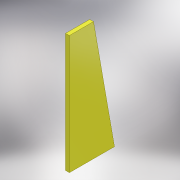
# Autodesk Inventor part: sides
Saved by Autodesk Inventor 2017 (Build 210142000, 142)
## iProperties
Created: 2017-03-04
Part Number: sides
Material: Acrylic
Document SubType Name: Modeling
Designer: dpgai
Density: 1.188 g/cm^3
Appearance: Yellow
Author: dpgai
Autodesk Inventor part; units mm, degrees
ref_plane "YZ Plane" through (0, 0, 0) normal (1, 0, 0) x (0, 1, 0)
ref_plane "XZ Plane" through (0, 0, 0) normal (0, 1, 0) x (-1, 0, 0)
ref_plane "XY Plane" through (0, 0, 0) normal (0, 0, 1) x (1, 0, 0)
sketch "Sketch1" plane through (0, 0, 0) normal (1, 0, 0) x (0, 1, 0)
  line L0 (0, 0) -> (20, 0)
  line L1 (20, 0) -> (37.3648, -98.4808)
  line L2 (37.3648, -98.4808) -> (0, -98.4808)
  line L3 (0, -98.4808) -> (0, 0)
  dimension "d0" = 20
  dimension "d1" = 100
  dimension "d4" = 98.4808
  dimension "d5" = 100
  constraints: 8 end point, 1 horizontal, 1 parallel, 1 perpendicular
  measures "d0" distance of L0.start L0.end
  measures "d1" distance of L0.end L1.end
  measures "d4" distance of L2.end L0.start
  measures "d5" angle of L0 L1
extrude "Extrusion1" add sketch "Sketch1" along normal blind 3.175
body "Solid1"
